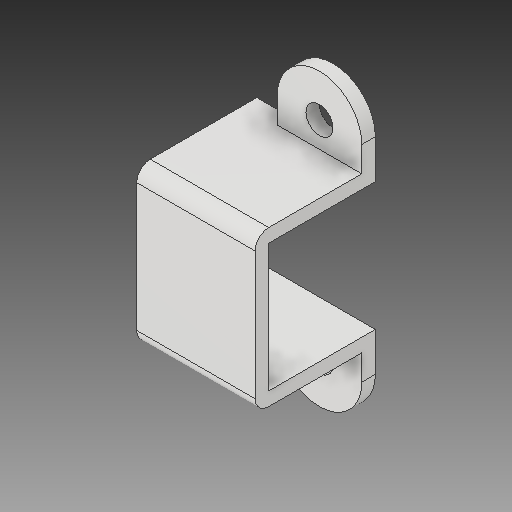
# Autodesk Inventor part: Mount
Saved by Autodesk Inventor 2017 (Build 210142000, 142)
## iProperties
Created: 2018-02-23
Part Number: Mount
Material: PAEK Plastic
Document SubType Name: Modeling
Designer: bradl
Density: 1.32 g/cm^3
Appearance: Smooth - White
Author: bradl
Autodesk Inventor part; units mm, degrees
ref_plane "YZ Plane" through (0, 0, 0) normal (1, 0, 0) x (0, 1, 0)
ref_plane "XZ Plane" through (0, 0, 0) normal (0, 1, 0) x (-1, 0, 0)
ref_plane "XY Plane" through (0, 0, 0) normal (0, 0, 1) x (1, 0, 0)
sketch "Sketch1" plane through (0, 0, 0) normal (1, 0, 0) x (0, 1, 0)
  arc A0 (4.3225, -9.9221) -> (5.9696, -5.6989) centre (-2.06, -5) ccw projected
  arc A1 (5.9244, -3.8989) -> (4.3225, -0.0779) centre (-2.06, -5) ccw projected
  arc A2 (-5.9696, -5.6989) -> (-4.3225, -9.9221) centre (2.06, -5) ccw projected
  arc A3 (-4.3225, -0.0779) -> (-5.9244, -3.8989) centre (2.06, -5) ccw projected
  line L0 (4.1641, 0) -> (-4.1641, 0) projected
  line L1 (-4.1641, -10) -> (4.1641, -10) projected
  line L2 (6, -10) -> (6, 0)
  line L3 (6, 0) -> (-6, 0)
  line L4 (-6, 0) -> (-6, -10)
  line L5 (-6, -10) -> (-7.27, -10)
  line L6 (-7.27, -10) -> (-7.27, 1.27)
  line L7 (6, -10) -> (7.27, -10)
  line L8 (6, 0) -> (6, 1.27) construction
  line L9 (6, 1.27) -> (-7.27, 1.27)
  line L10 (7.27, -10) -> (7.27, 1.27)
  line L11 (7.27, 1.27) -> (6, 1.27)
  point P0 (0, 0)
  dimension "d0" = 1.27
  dimension "d1" = 1.27
  dimension "d2" = 1.27
  constraints: 20 end point, 6 perpendicular, 3 point on line, 2 vertical, 1 horizontal
  measures "d0" distance of L4.end L5.end
  measures "d1" distance of L2.start L7.end
  measures "d2" distance of L2.end L8.end
extrude "Extrusion1" add sketch "Sketch1" along normal blind 11.1125
sketch "Sketch2" plane through (0, 7.27, 1.27) normal (0, 1, 0) x (1, 0, 0)
  line L0 (11.1125, 11.27) -> (11.1125, 0) projected
  line L1 (0, 11.27) -> (11.1125, 11.27) projected
  line L2 (0, 0) -> (0, 11.27) projected
  line L3 (11.1125, 11.27) -> (3.175, 11.27)
  line L4 (0, 11.27) -> (11.1125, 11.27) projected
  line L5 (3.175, 11.27) -> (3.175, 10)
  line L6 (3.175, 10) -> (11.1125, 10)
  point P0 (0, 1.27)
  dimension "d5" = 7.9375
  dimension "d6" = 1.27
  constraints: 6 end point, 2 perpendicular, 2 point on line
  measures "d5" distance of L0.start L3.end
  measures "d6" distance of L3.end L5.end
extrude "Extrusion2" add sketch "Sketch2" along normal blind 6.35
fillet "Fillet1" radius 3.9688 1 edges at (11.1125, 13.62, -9.365)
fillet "Fillet2" radius 3.9688 1 edges at (3.175, 13.62, -9.365)
sketch "Sketch3" plane through (3.175, 7.27, -8.73) normal (0, 0, 1) x (1, 0, 0)
  arc A0 (7.9375, 2.3812) -> (0, 2.3813) centre (3.9688, 2.3812) ccw projected
  line L0 (0, 0) -> (0, 2.3813) projected
  line L1 (7.9375, 0) -> (0, 0) projected
  line L2 (7.9375, 0) -> (7.9375, 2.3812) projected
  circle A1 centre (3.9688, 2.3812) radius 1.27
  point P0 (-3.175, -7.27)
  dimension "d11" = 2.54
  constraints: 1 centre point, 1 coincident
  measures "d11" diameter of A1
hole "Hole1" at (7.1438, 9.6513, -8.73) direction (0, 0, -1) diameter 2.54 end through all
sketch "Sketch4" plane through (0, -7.27, -10) normal (0, -1, 0) x (1, 0, 0)
  line L0 (0, 0) -> (0, 11.27) projected
  line L1 (0, 0) -> (11.1125, 0) projected
  line L2 (11.1125, 11.27) -> (11.1125, 0) projected
  line L3 (0, 11.27) -> (11.1125, 11.27) projected
  line L4 (0, 0) -> (11.1125, 0) projected
  line L5 (11.1125, 0) -> (3.175, 0)
  line L6 (11.1125, 1.27) -> (3.175, 1.27) projected
  line L7 (3.175, 0) -> (3.175, 1.27)
  line L8 (3.175, 1.27) -> (11.1125, 1.27)
  line L9 (11.1125, 1.27) -> (11.1125, 0) projected
  line L10 (11.1125, 1.27) -> (11.1125, 0)
  point P0 (0, 10)
  dimension "d19" = 7.9375
  dimension "d20" = 1.27
  constraints: 8 end point, 1 collinear, 1 point on line, 1 vertical
  measures "d19" distance of L1.end L5.end
  measures "d20" distance of L5.end L6.end
extrude "Extrusion3" add sketch "Sketch4" along normal blind 6.35 contours L7 L6 L2 L1
fillet "Fillet3" radius 3.9688 1 edges at (3.175, -13.62, -9.365)
fillet "Fillet4" radius 3.9688 1 edges at (11.1125, -13.62, -9.365)
sketch "Sketch5" plane through (3.175, -7.27, -8.73) normal (0, 0, 1) x (1, 0, 0)
  arc A0 (0, -2.3813) -> (7.9375, -2.3813) centre (3.9688, -2.3813) ccw projected
  line L0 (7.9375, 0) -> (7.9375, -2.3813) projected
  line L1 (0, 0) -> (7.9375, 0) projected
  line L2 (0, 0) -> (0, -2.3813) projected
  circle A1 centre (3.9688, -2.3813) radius 1.27
  point P0 (-3.175, 7.27)
  dimension "d25" = 2.54
  constraints: 1 centre point, 1 coincident
  measures "d25" diameter of A1
hole "Hole2" at (7.1438, -9.6513, -8.73) direction (0, 0, -1) diameter 2.54 end through all
fillet "Fillet5" radius 1.27 1 edges at (5.5563, -7.27, 1.27)
fillet "Fillet6" radius 1.27 1 edges at (5.5563, 7.27, 1.27)
body "Solid1"
